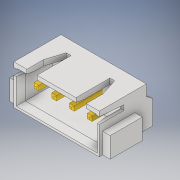
# Autodesk Inventor part: Nextion_Plug
Saved by Autodesk Inventor 2017 SP1 (Build 210196100, 196)
## iProperties
Created: 2016-08-29
Part Number: Nextion_Plug
Material: ABS Plastic
Document SubType Name: Modeling
Designer: jwrjc
Density: 1.06 g/cm^3
Appearance: Smooth - White
Author: jwrjc
Autodesk Inventor part; units mm, degrees
ref_plane "YZ Plane" through (0, 0, 0) normal (1, 0, 0) x (0, 1, 0)
ref_plane "XZ Plane" through (0, 0, 0) normal (0, 1, 0) x (-1, 0, 0)
ref_plane "XY Plane" through (0, 0, 0) normal (0, 0, 1) x (1, 0, 0)
sketch "Sketch1" plane through (0, 0, 0) normal (0, 0, 1) x (1, 0, 0)
  line L0 (6.4839, 37.011) -> (-6.0161, 37.011)
  line L1 (-6.0161, 37.011) -> (-6.0161, 29.211)
  line L2 (-6.0161, 29.211) -> (6.4839, 29.211)
  line L3 (6.4839, 29.211) -> (6.4839, 37.011)
  line L4 (7.5839, 36.511) -> (6.4839, 36.511)
  line L5 (6.4839, 36.511) -> (6.4839, 31.811)
  line L6 (6.4839, 31.811) -> (7.5839, 31.811)
  line L7 (7.5839, 31.811) -> (7.5839, 36.511)
  line L8 (-6.0161, 36.511) -> (-7.1161, 36.511)
  line L9 (-7.1161, 36.511) -> (-7.1161, 31.811)
  line L10 (-7.1161, 31.811) -> (-6.0161, 31.811)
  line L11 (-6.0161, 31.811) -> (-6.0161, 36.511)
  point P0 (0, 0)
  dimension "d0" = 12.5
  dimension "d1" = 7.8
  dimension "d2" = 1.1
  dimension "d3" = 4.7
  dimension "d4" = 1.1
  dimension "d5" = 4.7
  dimension "d6" = 0.5
  dimension "d7" = 0.5
  constraints: 24 end point, 6 parallel, 3 horizontal, 3 perpendicular, 2 collinear
  measures "d0" distance of L2.end L1.end
  measures "d1" distance of L1.end L0.end
  measures "d2" distance of L6.end L5.end
  measures "d3" distance of L5.end L4.end
  measures "d4" distance of L10.end L9.end
  measures "d5" distance of L9.end L8.end
  measures "d6" distance between parallel lines of L0 L4
  measures "d7" distance between parallel lines of L0 L8
extrude "Extrusion1" add sketch "Sketch1" along normal blind 5.8 contours L3 L2 L1 L0
extrude "Extrusion2" add sketch "Sketch1" along normal blind 3 contours L4 L7 L6 L3 | L1 L10 L9 L8
sketch "Sketch2" plane through (-6.0161, 37.011, 0) normal (0, 1, 0) x (1, 0, 0)
  line L0 (11.7, -5) -> (0.7, -5)
  line L1 (0.7, -5) -> (0.7, -0.8)
  line L2 (0.7, -0.8) -> (11.7, -0.8)
  line L3 (11.7, -0.8) -> (11.7, -5)
  line L4 (12.5, -5.8) -> (0, -5.8) projected
  line L5 (12.5, 0) -> (12.5, -5.8) projected
  point P0 (6.0161, 0)
  dimension "d12" = 11
  dimension "d13" = 4.2
  dimension "d14" = 0.8
  dimension "d15" = 0.8
  constraints: 8 end point, 2 parallel, 1 horizontal, 1 perpendicular
  measures "d12" distance of L1.end L2.end
  measures "d13" distance of L0.end L1.end
  measures "d14" distance between parallel lines of L0 L4
  measures "d15" distance between parallel lines of L3 L5
extrude "Extrusion3" cut sketch "Sketch2" against normal blind 5.1
move faces "Move1" translate (-0.25, 0, 0) faces at (-5.3161, 33.611, 3.6)
move faces "Move2" translate (0.25, 0, 0) faces at (5.6839, 35.311, 2.2)
move faces "Move3" translate (0, 0, -0.25) faces at (-1.7328, 35.311, 0.8)
sketch "Sketch3" plane through (0, 0, 5.8) normal (0, 0, 1) x (1, 0, 0)
  line L0 (3.0839, 37.011) -> (3.0839, 32.0463)
  line L1 (3.0839, 32.0463) -> (3.7839, 32.0463)
  line L2 (3.7839, 32.0463) -> (4.5839, 34.5287)
  line L3 (4.5839, 34.5287) -> (4.5839, 37.011)
  line L4 (4.5839, 37.011) -> (3.0839, 37.011)
  line L5 (6.4839, 37.011) -> (-6.0161, 37.011) projected
  line L6 (-2.6161, 37.011) -> (-2.6161, 32.0463)
  line L7 (-2.6161, 32.0463) -> (-3.3161, 32.0463)
  line L8 (-3.3161, 32.0463) -> (-4.1161, 34.5704)
  line L9 (-4.1161, 34.5704) -> (-4.1161, 37.011)
  line L10 (-2.6161, 37.011) -> (-4.1161, 37.011)
  line L11 (6.4839, 29.211) -> (6.4839, 37.011) projected
  line L12 (-6.0161, 37.011) -> (-6.0161, 29.211) projected
  point P0 (0, 0)
  dimension "d27" = 3.4
  dimension "d28" = 3.4
  dimension "d29" = 1.5
  dimension "d30" = 1.5
  dimension "d31" = 0.7
  dimension "d32" = 0.7
  constraints: 20 end point, 4 point on line, 3 perpendicular, 2 parallel, 1 collinear, 1 vertical
  measures "d27" distance between parallel lines of L0 L11
  measures "d28" distance between parallel lines of L6 L12
  measures "d29" distance between parallel lines of L0 L3
  measures "d30" distance between parallel lines of L9 L6
  measures "d31" distance of L0.end L1.end
  measures "d32" distance of L6.end L7.end
extrude "Extrusion4" cut sketch "Sketch3" against normal blind 1
sketch "Sketch4" plane through (-6.0161, 29.211, 5.8) normal (-1, 0, 0) x (0, 0, 1)
  line L0 (-5.8, 7.8) -> (0, 7.8) projected
  line L1 (-1.7, 7.8) -> (-1.7, 4.2)
  line L2 (-1.7, 4.2) -> (-1, 4.2)
  line L3 (-1, 4.2) -> (-0.8, 6.6699)
  line L4 (-0.8, 6.6699) -> (-0.8, 7.8)
  line L5 (-0.8, 7.8) -> (-1.7, 7.8)
  line L6 (0, 7.8) -> (0, 0) projected
  line L7 (0, 0.9) -> (-1.6, 0.9)
  line L8 (-1.6, 0.9) -> (-2.3, 0)
  line L9 (-2.3, 0) -> (0, 0)
  point P0 (-5.8, -29.211)
  dimension "d35" = 3.6
  dimension "d36" = 0.9
  dimension "d37" = 0.7
  dimension "d38" = 1.7
  dimension "d41" = 1.6
  dimension "d42" = 2.3
  dimension "d43" = 0.9
  constraints: 16 end point, 3 perpendicular, 3 point on line, 2 parallel, 1 vertical
  measures "d35" distance between parallel lines of L2 L0
  measures "d36" distance between parallel lines of L1 L4
  measures "d37" distance of L1.end L2.end
  measures "d38" distance between parallel lines of L1 L6
  measures "d41" distance of L7.start L7.end
  measures "d42" distance of L8.end L6.end
  measures "d43" distance between parallel lines of L9 L7
extrude "Extrusion5" cut sketch "Sketch4" against normal blind 12.75
sketch "Sketch5" plane through (-6.0161, 29.211, 0) normal (0, -1, 0) x (1, 0, 0)
  line L0 (11.95, 5) -> (0.45, 5) projected
  line L1 (0.45, 5) -> (0.45, 0.55) projected
  line L2 (0.45, 0.55) -> (11.95, 0.55) projected
  line L3 (11.95, 0.55) -> (11.95, 5) projected
  point P0 (6.0161, 0)
extrude "Extrusion6" cut sketch "Sketch5" against normal blind 1.25
ref_plane "Work Plane1" through (-6.0161, 36.261, 0) normal (0, 1, 0) x (1, 0, 0)
sketch "Sketch6" plane through (-6.0161, 36.261, 0) normal (0, 1, 0) x (1, 0, 0)
  line L0 (10.5, -3.7) -> (9.8, -3.7)
  line L1 (9.8, -3.7) -> (9.8, -3)
  line L2 (9.8, -3) -> (10.5, -3)
  line L3 (10.5, -3) -> (10.5, -3.7)
  line L4 (7.9, -3.7) -> (7.2, -3.7)
  line L5 (7.2, -3.7) -> (7.2, -3)
  line L6 (7.2, -3) -> (7.9, -3)
  line L7 (7.9, -3) -> (7.9, -3.7)
  line L8 (5.3, -3.7) -> (4.6, -3.7)
  line L9 (4.6, -3.7) -> (4.6, -3)
  line L10 (4.6, -3) -> (5.3, -3)
  line L11 (5.3, -3) -> (5.3, -3.7)
  line L12 (2.7, -3.7) -> (2, -3.7)
  line L13 (2, -3.7) -> (2, -3)
  line L14 (2, -3) -> (2.7, -3)
  line L15 (2.7, -3) -> (2.7, -3.7)
  line L16 (0, 0) -> (0, -4.1) projected
  line L17 (12.5, 0) -> (12.5, -4.1) projected
  line L18 (12.5, -5) -> (10.6, -5) projected
  point P0 (6.0161, 0)
  dimension "d47" = 0.7
  dimension "d48" = 0.7
  dimension "d49" = 0.7
  dimension "d50" = 0.7
  dimension "d51" = 0.7
  dimension "d52" = 0.7
  dimension "d53" = 0.7
  dimension "d54" = 2.7
  dimension "d55" = 2.7
  dimension "d56" = 1.9
  dimension "d57" = 1.9
  dimension "d58" = 1.9
  dimension "d59" = 1.3
  constraints: 32 end point, 8 parallel, 4 horizontal, 4 perpendicular, 4 point on line
  measures "d47" distance of L1.end L2.end
  measures "d48" distance of L0.end L1.end
  measures "d49" distance of L5.end L6.end
  measures "d50" distance of L4.end L5.end
  measures "d51" distance of L9.end L10.end
  measures "d52" distance of L8.end L9.end
  measures "d53" distance of L13.end L14.end
  measures "d54" distance between parallel lines of L16 L15
  measures "d55" distance between parallel lines of L17 L1
  measures "d56" distance between parallel lines of L7 L1
  measures "d57" distance between parallel lines of L15 L9
  measures "d58" distance between parallel lines of L11 L5
  measures "d59" distance between parallel lines of L18 L0
extrude "Extrusion7" add sketch "Sketch6" against normal blind 11.6 separate body
sketch "Sketch7" plane through (0, 0, 0) normal (0, 0, -1) x (-1, 0, 0)
  line L0 (-5.9339, 30.461) -> (5.5661, 30.461) projected
  line L1 (6.0161, 29.211) -> (-6.4839, 29.211) projected
  line L2 (4.2092, 29.211) -> (3.113, 29.211)
  line L3 (3.113, 29.211) -> (3.113, 30.461)
  line L4 (3.113, 30.461) -> (4.2092, 30.461)
  line L5 (4.2092, 30.461) -> (4.2092, 29.211)
  line L6 (1.603, 29.211) -> (0.5274, 29.211)
  line L7 (0.5274, 29.211) -> (0.5274, 30.461)
  line L8 (0.5274, 30.461) -> (1.603, 30.461)
  line L9 (1.603, 30.461) -> (1.603, 29.211)
  line L10 (5.5661, 30.461) -> (-5.9339, 30.461) projected
  line L11 (-0.9825, 29.211) -> (-2.0995, 29.211)
  line L12 (-2.0995, 29.211) -> (-2.0995, 30.461)
  line L13 (-2.0995, 30.461) -> (-0.9825, 30.461)
  line L14 (-0.9825, 30.461) -> (-0.9825, 29.211)
  line L15 (-3.6094, 29.211) -> (-4.685, 29.211)
  line L16 (-4.685, 29.211) -> (-4.685, 30.461)
  line L17 (-4.685, 30.461) -> (-3.6094, 30.461)
  line L18 (-3.6094, 30.461) -> (-3.6094, 29.211)
  point P0 (0, 0)
  constraints: 32 end point, 8 parallel, 8 point on line, 4 horizontal, 4 perpendicular
extrude "Extrusion8" cut sketch "Sketch7" against normal blind 0.65 contours L0 L18 L1 L16 | L0 L14 L1 L12 | L0 L9 L1 L7 | L0 L5 L1 L3 bodies 1
move faces "Move4" translate (0, 4.25, 0) faces at (-3.5495, 24.661, 3.4667) (-1.1828, 24.661, 3.2333) (1.6505, 24.661, 3.4667) (4.2505, 24.661, 3.4667)
move faces "Move5" translate (0, 0.5, 0) faces at (4.2505, 28.911, 3.4667) (1.6505, 28.911, 3.4667) (-1.1828, 28.911, 3.2333) (-3.5495, 28.911, 3.4667)
sketch "Sketch8" plane through (4.4839, 36.261, 3) normal (0, 0, -1) x (-1, 0, 0)
  line L0 (0.7, 0) -> (0.7, -6.85) projected
  line L1 (10.05, -6.15) -> (-1.45, -6.15) projected
  line L2 (0.7, -6.85) -> (0, -6.85)
  line L3 (0, -6.85) -> (0, -6.15)
  line L4 (0, -6.15) -> (0.7, -6.15)
  line L5 (0.7, -6.15) -> (0.7, -6.85)
  line L6 (2.6, -6.85) -> (3.3, -6.85) projected
  line L7 (3.3, -6.85) -> (2.6, -6.85)
  line L8 (2.6, -6.85) -> (2.6, -6.15)
  line L9 (2.6, -6.15) -> (3.3, -6.15)
  line L10 (3.3, -6.15) -> (3.3, -6.85)
  line L11 (5.9, -6.85) -> (5.2, -6.85)
  line L12 (5.2, -6.85) -> (5.2, -6.15)
  line L13 (5.2, -6.15) -> (5.9, -6.15)
  line L14 (5.9, -6.15) -> (5.9, -6.85)
  line L15 (8.5, -6.85) -> (7.8, -6.85) projected
  line L16 (8.5, -6.85) -> (7.8, -6.85)
  line L17 (7.8, -6.85) -> (7.8, -6.15)
  line L18 (7.8, -6.15) -> (8.5, -6.15)
  line L19 (8.5, -6.15) -> (8.5, -6.85)
  line L20 (5.9, 0) -> (5.9, -6.85) projected
  point P0 (4.4839, -36.261)
  dimension "d70" = 0.7
  dimension "d71" = 0.7
  dimension "d72" = 0.7
  dimension "d73" = 0.7
  dimension "d74" = 0.7
  dimension "d75" = 0.7
  constraints: 32 end point, 8 parallel, 4 horizontal, 4 perpendicular, 3 point on line, 1 collinear
  measures "d70" distance of L3.end L4.end
  measures "d71" distance of L8.end L9.end
  measures "d72" distance of L7.end L8.end
  measures "d73" distance of L12.end L13.end
  measures "d74" distance of L17.end L18.end
  measures "d75" distance of L16.end L17.end
extrude "Extrusion9" add sketch "Sketch8" along normal blind 2.98 bodies 2
sketch "Sketch9" plane through (-4.0161, 29.411, 3.7) normal (0, -1, 0) x (1, 0, 0)
  line L0 (0, 0) -> (0, -3.68) projected
  line L1 (0, -3.68) -> (0.7, -3.68)
  line L2 (0.7, -3.68) -> (0.7, -2.98)
  line L3 (0.7, -2.98) -> (0, -2.98)
  line L4 (0, -2.98) -> (0, -3.68)
  line L5 (2.5963, -0.7) -> (2.5963, -3.68) projected
  line L6 (2.6, -3.68) -> (3.3, -3.68)
  line L7 (3.3, -3.68) -> (3.3, -2.98)
  line L8 (3.3, -2.98) -> (2.6, -2.98)
  line L9 (2.6, -2.98) -> (2.6, -3.68)
  line L10 (5.2, -0.7) -> (5.2, -3.68) projected
  line L11 (5.2, -3.68) -> (5.9, -3.68)
  line L12 (5.9, -3.68) -> (5.9, -2.98)
  line L13 (5.9, -2.98) -> (5.2, -2.98)
  line L14 (5.2, -2.98) -> (5.2, -3.68)
  line L15 (7.8, 0) -> (7.8, -3.68) projected
  line L16 (7.8, -3.68) -> (8.5, -3.68)
  line L17 (8.5, -3.68) -> (8.5, -2.98)
  line L18 (8.5, -2.98) -> (7.8, -2.98)
  line L19 (7.8, -2.98) -> (7.8, -3.68)
  point P0 (4.0161, -3.7)
  point P1 (2.6193, -0.7)
  dimension "d78" = 0.7
  dimension "d79" = 0.7
  dimension "d80" = 0.7
  dimension "d81" = 0.7
  dimension "d82" = 0.7
  dimension "d83" = 0.7
  dimension "d84" = 0.7
  dimension "d85" = 0.7
  constraints: 32 end point, 8 parallel, 4 horizontal, 4 perpendicular, 1 other
  measures "d78" distance of L3.end L2.end
  measures "d79" distance of L2.end L1.end
  measures "d80" distance of L8.end L7.end
  measures "d81" distance of L7.end L6.end
  measures "d82" distance of L13.end L12.end
  measures "d83" distance of L12.end L11.end
  measures "d84" distance of L18.end L17.end
  measures "d85" distance of L17.end L16.end
extrude "Extrusion10" add sketch "Sketch9" along normal blind 2.2 bodies 2
fillet "Fillet1" radius 0.4 16 edges at (-3.6661, 29.411, 3.7) (-1.0661, 29.411, 3.7) (1.5339, 29.411, 3.7) (4.1339, 29.411, 3.7) (4.1339, 30.111, 3) (1.5339, 30.111, 3) (-1.0661, 30.111, 3) (-3.6661, 30.111, 3) (-3.6661, 29.411, 0.72) (-1.0661, 29.411, 0.72) (1.5339, 29.411, 0.72) (4.1339, 29.411, 0.72) (-3.6661, 30.111, 0.02) (-1.0661, 30.111, 0.02) (1.5339, 30.111, 0.02) (4.1339, 30.111, 0.02)
chamfer "Chamfer1" distance 0.2 angle 45 16 edges at (4.1339, 36.261, 3.7) (3.7839, 36.261, 3.35) (4.1339, 36.261, 3) (4.4839, 36.261, 3.35) (1.8839, 36.261, 3.35) (1.5339, 36.261, 3.7) (1.1839, 36.261, 3.35) (1.5339, 36.261, 3) (-0.7161, 36.261, 3.35) (-1.0661, 36.261, 3.7) (-1.4161, 36.261, 3.35) (-1.0661, 36.261, 3) (-3.3161, 36.261, 3.35) (-3.6661, 36.261, 3.7) (-4.0161, 36.261, 3.35) (-3.6661, 36.261, 3)
chamfer "Chamfer2" distance 0.2 angle 80 3 edges at (5.9339, 37.011, 2.325) (0.1839, 37.011, 0.55) (-5.5661, 37.011, 2.325) measured on face at (0.1839, 37.011, 0.45) measured on face at (-5.6661, 37.011, 2.325) measured on face at (6.0339, 37.011, 2.325)
chamfer "Chamfer3" distance 0.2 angle 80 1 edges at (5.5339, 37.011, 5) measured on face at (5.5339, 37.011, 5.5)
chamfer "Chamfer4" distance 0.2 angle 80 1 edges at (0.2339, 37.011, 5) measured on face at (0.2339, 37.011, 5.5)
chamfer "Chamfer5" distance 0.2 angle 80 1 edges at (-5.0661, 37.011, 5) measured on face at (-5.0661, 37.011, 5.5)
body "Solid1"
body "Solid2"
